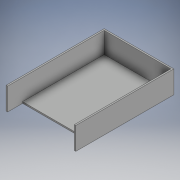
# Autodesk Inventor part: Component box top
Saved by Autodesk Inventor 2021 (Build 250183000, 183)
## iProperties
Created: 2023-01-12
Part Number: Component box top
Material: Generic
Document SubType Name: Modeling
Designer: boyle
Density: 1 g/cm^3
Appearance: Default
Author: boyle
Autodesk Inventor part; units mm, degrees
ref_plane "YZ Plane" through (0, 0, 0) normal (1, 0, 0) x (0, 1, 0)
ref_plane "XZ Plane" through (0, 0, 0) normal (0, 1, 0) x (-1, 0, 0)
ref_plane "XY Plane" through (0, 0, 0) normal (0, 0, 1) x (1, 0, 0)
sketch "Sketch1" plane through (0, 0, 0) normal (0, 1, 0) x (-1, 0, 0)
  line L0 (0, 0) -> (-177.8, 0)
  line L1 (-177.8, 0) -> (-177.8, 254)
  line L2 (-177.8, 254) -> (0, 254)
  line L3 (0, 254) -> (0, 0)
  dimension "d0" = 177.8
  dimension "d1" = 254
  constraints: 8 end point, 2 parallel, 1 horizontal, 1 perpendicular
  measures "d0" distance of L1.end L2.end
  measures "d1" distance of L0.end L1.end
extrude "Extrusion1" add sketch "Sketch1" along normal blind 57.15
shell "Shell1" thickness 3.81 removed faces 1 at (118.5333, 57.15, 169.3333)
sketch "Sketch2" plane through (0, 0, 254) normal (0, 0, 1) x (1, 0, 0)
  line L0 (0, 0) -> (177.8, 0) projected
  line L1 (177.8, 0) -> (177.8, 57.15) projected
  line L2 (0, 57.15) -> (177.8, 57.15) projected
  line L3 (0, 0) -> (0, 57.15) projected
extrude "Extrusion2" cut sketch "Sketch2" against normal up to surface (3.81 mm away)
sketch "Sketch3" plane through (3.81, 3.81, 3.81) normal (0, 1, 0) x (1, 0, 0)
  line L0 (0, -246.38) -> (170.18, -246.38) projected
  line L1 (170.18, -246.38) -> (170.18, 0) projected
  line L2 (0, 0) -> (0, -246.38) projected
  line L3 (170.18, -246.38) -> (-1.2603, -246.38)
  line L4 (-1.2603, -246.38) -> (-1.2603, -208.28)
  line L5 (-1.2603, -208.28) -> (170.18, -208.28)
  line L6 (170.18, -208.28) -> (170.18, -246.38)
  point P0 (-3.81, 3.81)
  point P1 (0, -208.28)
  dimension "d7" = 38.1
  constraints: 8 end point, 2 parallel, 1 horizontal, 1 perpendicular
  measures "d7" distance of L3.end L4.end
extrude "Extrusion3" cut sketch "Sketch3" against normal through all contours L2 L5 L1 L0
body "Solid1"
